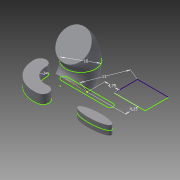
# Autodesk Inventor part: Demo-Status-0.2
Saved by Autodesk Inventor 2015 (Build 190159000, 159)
## iProperties
Created: 2017-04-06
Part Number: Demo-Status-0.2
Material: Generisch
Document SubType Name: Modeling
Designer: jensp
Density: 1 g/cm^3
Appearance: Vorgabe
Author: jensp
Autodesk Inventor part; units mm, degrees
ref_plane "YZ Plane" through (0, 0, 0) normal (1, 0, 0) x (0, 1, 0)
ref_plane "XZ Plane" through (0, 0, 0) normal (0, 1, 0) x (-1, 0, 0)
ref_plane "XY Plane" through (0, 0, 0) normal (0, 0, 1) x (1, 0, 0)
sketch "Demo-Sketch-01" plane through (0, 0, 0) normal (0, 0, 1) x (1, 0, 0)
  circle A0 centre (-10.3253, 8.1356) radius 5
  line L0 (4.75, 4.25) -> (15.1674, 4.25)
  line L1 (15.1674, 4.25) -> (15.1674, 12.1011)
  line L2 (15.1674, 12.1011) -> (4.75, 12.1011)
  line L3 (4.75, 12.1011) -> (4.75, 4.25)
  ellipse E0 centre (9.6666, -7.1387) end of major axis (15.1674, -6.9606) minor radius 1.5371
  line L4 (-7.7973, 0) -> (7.6193, 0) construction
  line L5 (-7.7973, -1.0147) -> (7.6193, -1.0147)
  line L6 (7.6193, 1.0147) -> (-7.7973, 1.0147)
  arc A1 (-7.7973, 1.0147) -> (-7.7973, -1.0147) centre (-7.7973, 0) ccw
  arc A2 (7.6193, -1.0147) -> (7.6193, 1.0147) centre (7.6193, 0) ccw
  arc A3 (-13.2422, -2.4939) -> (-5.2363, -9.673) centre (-6.2467, -2.7463) ccw construction
  arc A4 (-15.2409, -2.4218) -> (-4.9476, -11.6521) centre (-6.2467, -2.7463) ccw
  arc A5 (-11.2435, -2.566) -> (-5.525, -7.6939) centre (-6.2467, -2.7463) ccw
  arc A6 (-11.2435, -2.566) -> (-15.2409, -2.4218) centre (-13.2422, -2.4939) ccw
  arc A7 (-4.9476, -11.6521) -> (-5.525, -7.6939) centre (-5.2363, -9.673) ccw
  point P0 (0, 0)
  point P1 (-0.089, 0)
  dimension "d0" = 10
  dimension "d1" = 2
  dimension "d2" = 4.25
  dimension "d3" = 13
  dimension "d4" = 4.75
  constraints: 16 end point, 14 point on circle, 8 centre point, 8 tangent, 3 parallel, 2 horizontal, 1 equal radius, 1 midpoint, 1 perpendicular, 2 other
  measures "d0" diameter of A0
  measures "d1" radius of A6
  measures "d2" vertical distance of point (-0.089, 0) L0.start
  measures "d3" distance of point (0, 0) L2.end
  measures "d4" horizontal distance of point (0, 0) L0.start
extrude "Extrusion1" add sketch "Demo-Sketch-01" along normal blind 3 contours A6 A5 A7 A4
extrude "Extrusion2" add sketch "Demo-Sketch-01" along normal mid plane 3 contours E0
revolve "Umdrehung1" add sketch "Demo-Sketch-01" angle 90 mid plane about axis through (-7.7973, 0, 0) along (1, 0, 0) contours A0
